Autodesk Inventor part; units mm, degrees
(part 4 of 6)
  line L1347 (22.7558, -15.0073) -> (22.7978, -15.0253) construction
  line L1348 (22.7978, -15.0253) -> (23.0138, -14.7074) construction
  line L1349 (23.0138, -14.7074) -> (23.0378, -14.6833) construction
  spline S408 degree 3 poles (23.0378, -14.6833) (23.0798, -14.6113) (23.1218, -14.5333) (23.1698, -14.4614) knots 110 110 110 110 111 111 111 111
  line L1350 (23.0378, -14.6833) -> (23.0798, -14.6113) construction
  line L1351 (23.0798, -14.6113) -> (23.1218, -14.5333) construction
  line L1352 (23.1218, -14.5333) -> (23.1698, -14.4614) construction
  spline S409 degree 3 poles (23.1698, -14.4614) (23.2118, -14.4073) (23.1998, -14.4134) (23.2598, -14.3894) knots 111 111 111 111 112 112 112 112
  line L1353 (23.1698, -14.4614) -> (23.2118, -14.4073) construction
  line L1354 (23.2118, -14.4073) -> (23.1998, -14.4134) construction
  line L1355 (23.1998, -14.4134) -> (23.2598, -14.3894) construction
  spline S410 degree 3 poles (23.2598, -14.3894) (23.2538, -14.3954) (23.3318, -14.3714) (23.3438, -14.3714) knots 112 112 112 112 113 113 113 113
  line L1356 (23.2598, -14.3894) -> (23.2538, -14.3954) construction
  line L1357 (23.2538, -14.3954) -> (23.3318, -14.3714) construction
  line L1358 (23.3318, -14.3714) -> (23.3438, -14.3714) construction
  spline S411 degree 3 poles (23.3438, -14.3714) (23.3799, -14.3648) (23.6063, -14.3474) (23.7756, -14.2966) knots 113 113 113 113 114 114 114 114
  line L1359 (23.3438, -14.3714) -> (23.3799, -14.3648) construction
  line L1360 (23.3799, -14.3648) -> (23.6063, -14.3474) construction
  line L1361 (23.6063, -14.3474) -> (23.7756, -14.2966) construction
  spline S412 degree 3 poles (23.7756, -14.2966) (23.7091, -14.4879) (23.6088, -14.7871) (23.6258, -14.7913) knots 114 114 114 114 115 115 115 115
  line L1362 (23.7756, -14.2966) -> (23.7091, -14.4879) construction
  line L1363 (23.7091, -14.4879) -> (23.6088, -14.7871) construction
  line L1364 (23.6088, -14.7871) -> (23.6258, -14.7913) construction
  spline S413 degree 3 poles (23.6258, -14.7913) (23.6258, -14.7913) (23.6378, -14.7853) (23.6378, -14.7794) knots 115 115 115 115 116 116 116 116
  line L1365 (23.6258, -14.7913) -> (23.6258, -14.7913) construction
  line L1366 (23.6258, -14.7913) -> (23.6378, -14.7853) construction
  line L1367 (23.6378, -14.7853) -> (23.6378, -14.7794) construction
  spline S414 degree 3 poles (23.6378, -14.7794) (23.6258, -14.8153) (23.6198, -14.8633) (23.6138, -14.9054) knots 116 116 116 116 117 117 117 117
  line L1368 (23.6378, -14.7794) -> (23.6258, -14.8153) construction
  line L1369 (23.6258, -14.8153) -> (23.6198, -14.8633) construction
  line L1370 (23.6198, -14.8633) -> (23.6138, -14.9054) construction
  spline S415 degree 3 poles (23.6138, -14.9054) (23.6018, -14.9054) (23.6198, -14.8693) (23.6078, -14.8693) knots 117 117 117 117 118 118 118 118
  line L1371 (23.6138, -14.9054) -> (23.6018, -14.9054) construction
  line L1372 (23.6018, -14.9054) -> (23.6198, -14.8693) construction
  line L1373 (23.6198, -14.8693) -> (23.6078, -14.8693) construction
  spline S416 degree 3 poles (23.6078, -14.8693) (23.5718, -14.8633) (23.5238, -15.1693) (23.5238, -15.1813) knots 118 118 118 118 119 119 119 119
  line L1374 (23.6078, -14.8693) -> (23.5718, -14.8633) construction
  line L1375 (23.5718, -14.8633) -> (23.5238, -15.1693) construction
  line L1376 (23.5238, -15.1693) -> (23.5238, -15.1813) construction
  spline S417 degree 3 poles (23.5238, -15.1813) (23.5178, -15.3013) (23.5478, -15.4153) (23.6018, -15.5173) knots 119 119 119 119 120 120 120 120
  line L1377 (23.5238, -15.1813) -> (23.5178, -15.3013) construction
  line L1378 (23.5178, -15.3013) -> (23.5478, -15.4153) construction
  line L1379 (23.5478, -15.4153) -> (23.6018, -15.5173) construction
  spline S418 degree 3 poles (23.6018, -15.5173) (23.6438, -15.5833) (23.6858, -15.6373) (23.7578, -15.6613) knots 120 120 120 120 121 121 121 121
  line L1380 (23.6018, -15.5173) -> (23.6438, -15.5833) construction
  line L1381 (23.6438, -15.5833) -> (23.6858, -15.6373) construction
  line L1382 (23.6858, -15.6373) -> (23.7578, -15.6613) construction
  spline S419 degree 3 poles (23.7578, -15.6613) (23.7998, -15.6793) (23.8478, -15.6853) (23.8958, -15.6793) knots 121 121 121 121 122 122 122 122
  line L1383 (23.7578, -15.6613) -> (23.7998, -15.6793) construction
  line L1384 (23.7998, -15.6793) -> (23.8478, -15.6853) construction
  line L1385 (23.8478, -15.6853) -> (23.8958, -15.6793) construction
  spline S420 degree 3 poles (23.8958, -15.6793) (23.9078, -15.6793) (24.0157, -15.6433) (23.9678, -15.6433) knots 122 122 122 122 123 123 123 123
  line L1386 (23.8958, -15.6793) -> (23.9078, -15.6793) construction
  line L1387 (23.9078, -15.6793) -> (24.0157, -15.6433) construction
  line L1388 (24.0157, -15.6433) -> (23.9678, -15.6433) construction
  line L1389 (23.9678, -15.6433) -> (24.0278, -15.6253)
  line L1390 (24.0278, -15.6253) -> (23.9918, -15.6433)
  spline S421 degree 3 poles (23.9918, -15.6433) (23.9978, -15.6493) (24.1658, -15.5653) (24.1898, -15.5593) knots 125 125 125 125 126 126 126 126
  line L1391 (23.9918, -15.6433) -> (23.9978, -15.6493) construction
  line L1392 (23.9978, -15.6493) -> (24.1658, -15.5653) construction
  line L1393 (24.1658, -15.5653) -> (24.1898, -15.5593) construction
  spline S422 degree 3 poles (24.1898, -15.5593) (24.3158, -15.5053) (24.4237, -15.4153) (24.5197, -15.3193) knots 126 126 126 126 127 127 127 127
  line L1394 (24.1898, -15.5593) -> (24.3158, -15.5053) construction
  line L1395 (24.3158, -15.5053) -> (24.4237, -15.4153) construction
  line L1396 (24.4237, -15.4153) -> (24.5197, -15.3193) construction
  spline S423 degree 3 poles (24.5197, -15.3193) (24.7057, -15.1213) (24.8677, -14.8813) (25.0357, -14.6593) knots 127 127 127 127 128 128 128 128
  line L1397 (24.5197, -15.3193) -> (24.7057, -15.1213) construction
  line L1398 (24.7057, -15.1213) -> (24.8677, -14.8813) construction
  line L1399 (24.8677, -14.8813) -> (25.0357, -14.6593) construction
  spline S424 degree 3 poles (25.0357, -14.6593) (25.0237, -14.7253) (24.8737, -15.4753) (24.9157, -15.4753) knots 128 128 128 128 129 129 129 129
  line L1400 (25.0357, -14.6593) -> (25.0237, -14.7253) construction
  line L1401 (25.0237, -14.7253) -> (24.8737, -15.4753) construction
  line L1402 (24.8737, -15.4753) -> (24.9157, -15.4753) construction
  line L1403 (24.9157, -15.4753) -> (24.9277, -15.4513)
  spline S425 degree 3 poles (24.9277, -15.4513) (24.9277, -15.5053) (24.9277, -15.5593) (24.9337, -15.6073) knots 130 130 130 130 131 131 131 131
  line L1404 (24.9277, -15.4513) -> (24.9277, -15.5053) construction
  line L1405 (24.9277, -15.5053) -> (24.9277, -15.5593) construction
  line L1406 (24.9277, -15.5593) -> (24.9337, -15.6073) construction
  spline S426 degree 3 poles (24.9337, -15.6073) (24.9217, -15.6073) (24.9277, -15.5653) (24.9157, -15.5653) knots 131 131 131 131 132 132 132 132
  line L1407 (24.9337, -15.6073) -> (24.9217, -15.6073) construction
  line L1408 (24.9217, -15.6073) -> (24.9277, -15.5653) construction
  line L1409 (24.9277, -15.5653) -> (24.9157, -15.5653) construction
  spline S427 degree 3 poles (24.9157, -15.5653) (24.8797, -15.5713) (24.9217, -15.8233) (24.9277, -15.8473) knots 132 132 132 132 133 133 133 133
  line L1410 (24.9157, -15.5653) -> (24.8797, -15.5713) construction
  line L1411 (24.8797, -15.5713) -> (24.9217, -15.8233) construction
  line L1412 (24.9217, -15.8233) -> (24.9277, -15.8473) construction
  spline S428 degree 3 poles (24.9277, -15.8473) (24.9577, -15.9493) (25.0057, -16.0513) (25.1017, -16.0993) knots 133 133 133 133 134 134 134 134
  line L1413 (24.9277, -15.8473) -> (24.9577, -15.9493) construction
  line L1414 (24.9577, -15.9493) -> (25.0057, -16.0513) construction
  line L1415 (25.0057, -16.0513) -> (25.1017, -16.0993) construction
  spline S429 degree 3 poles (25.1017, -16.0993) (25.1977, -16.1473) (25.3417, -16.1533) (25.4497, -16.1353) knots 134 134 134 134 135 135 135 135
  line L1416 (25.1017, -16.0993) -> (25.1977, -16.1473) construction
  line L1417 (25.1977, -16.1473) -> (25.3417, -16.1533) construction
  line L1418 (25.3417, -16.1533) -> (25.4497, -16.1353) construction
  spline S430 degree 3 poles (25.4497, -16.1353) (25.5217, -16.1233) (25.5997, -16.0933) (25.6597, -16.0453) knots 135 135 135 135 136 136 136 136
  line L1419 (25.4497, -16.1353) -> (25.5217, -16.1233) construction
  line L1420 (25.5217, -16.1233) -> (25.5997, -16.0933) construction
  line L1421 (25.5997, -16.0933) -> (25.6597, -16.0453) construction
  spline S431 degree 3 poles (25.6597, -16.0453) (25.6657, -16.0393) (25.7497, -15.9493) (25.7257, -15.9553) knots 136 136 136 136 137 137 137 137
  line L1422 (25.6597, -16.0453) -> (25.6657, -16.0393) construction
  line L1423 (25.6657, -16.0393) -> (25.7497, -15.9493) construction
  line L1424 (25.7497, -15.9493) -> (25.7257, -15.9553) construction
  line L1425 (25.7257, -15.9553) -> (25.7557, -15.9373)
  spline S432 degree 3 poles (25.7557, -15.9373) (25.7497, -15.9433) (25.7497, -15.9493) (25.7497, -15.9553) knots 138 138 138 138 139 139 139 139
  line L1426 (25.7557, -15.9373) -> (25.7497, -15.9433) construction
  line L1427 (25.7497, -15.9433) -> (25.7497, -15.9493) construction
  line L1428 (25.7497, -15.9493) -> (25.7497, -15.9553) construction
  spline S433 degree 3 poles (25.7497, -15.9553) (25.7557, -15.9613) (25.9357, -15.7693) (25.9597, -15.7513) knots 139 139 139 139 140 140 140 140
  line L1429 (25.7497, -15.9553) -> (25.7557, -15.9613) construction
  line L1430 (25.7557, -15.9613) -> (25.9357, -15.7693) construction
  line L1431 (25.9357, -15.7693) -> (25.9597, -15.7513) construction
  spline S434 degree 3 poles (25.9597, -15.7513) (26.0737, -15.6493) (26.1637, -15.4993) (26.2297, -15.3673) knots 140 140 140 140 141 141 141 141
  line L1432 (25.9597, -15.7513) -> (26.0737, -15.6493) construction
  line L1433 (26.0737, -15.6493) -> (26.1637, -15.4993) construction
  line L1434 (26.1637, -15.4993) -> (26.2297, -15.3673) construction
  line L1435 (26.2297, -15.3673) -> (26.3317, -15.1453)
  line L1436 (26.3317, -15.1453) -> (26.3797, -15.0253)
  spline S435 degree 3 poles (26.3797, -15.0253) (26.3977, -14.9953) (26.4097, -14.9654) (26.4217, -14.9353) knots 143 143 143 143 144 144 144 144
  line L1437 (26.3797, -15.0253) -> (26.3977, -14.9953) construction
  line L1438 (26.3977, -14.9953) -> (26.4097, -14.9654) construction
  line L1439 (26.4097, -14.9654) -> (26.4217, -14.9353) construction
  spline S436 degree 3 poles (26.4217, -14.9353) (26.4337, -14.9353) (26.4517, -14.9413) (26.4637, -14.9413) knots 144 144 144 144 145 145 145 145
  line L1440 (26.4217, -14.9353) -> (26.4337, -14.9353) construction
  line L1441 (26.4337, -14.9353) -> (26.4517, -14.9413) construction
  line L1442 (26.4517, -14.9413) -> (26.4637, -14.9413) construction
  spline S437 degree 3 poles (26.4637, -14.9413) (26.5837, -14.9173) (26.7037, -14.9594) (26.8237, -14.9173) knots 145 145 145 145 146 146 146 146
  line L1443 (26.4637, -14.9413) -> (26.5837, -14.9173) construction
  line L1444 (26.5837, -14.9173) -> (26.7037, -14.9594) construction
  line L1445 (26.7037, -14.9594) -> (26.8237, -14.9173) construction
  spline S438 degree 3 poles (26.8237, -14.9173) (27.0757, -14.8394) (27.2557, -14.6234) (27.4237, -14.4494) knots 146 146 146 146 147 147 147 147
  line L1446 (26.8237, -14.9173) -> (27.0757, -14.8394) construction
  line L1447 (27.0757, -14.8394) -> (27.2557, -14.6234) construction
  line L1448 (27.2557, -14.6234) -> (27.4237, -14.4494) construction
  spline S439 degree 3 poles (27.4237, -14.4494) (27.4717, -14.4013) (27.6337, -14.2694) (27.6217, -14.1734) knots 147 147 147 147 148 148 148 148
  line L1449 (27.4237, -14.4494) -> (27.4717, -14.4013) construction
  line L1450 (27.4717, -14.4013) -> (27.6337, -14.2694) construction
  line L1451 (27.6337, -14.2694) -> (27.6217, -14.1734) construction
  spline S440 degree 3 poles (27.6217, -14.1734) (27.6097, -14.0474) (27.4657, -14.1014) (27.3997, -14.1434) knots 148 148 148 148 149 149 149 149
  line L1452 (27.6217, -14.1734) -> (27.6097, -14.0474) construction
  line L1453 (27.6097, -14.0474) -> (27.4657, -14.1014) construction
  line L1454 (27.4657, -14.1014) -> (27.3997, -14.1434) construction
  spline S441 degree 3 poles (22.6358, -13.2434) (22.6358, -13.2494) (22.6298, -13.2494) (22.6298, -13.2494) knots 0 0 0 0 1 1 1 1
  line L1455 (22.6358, -13.2434) -> (22.6358, -13.2494) construction
  line L1456 (22.6358, -13.2494) -> (22.6298, -13.2494) construction
  line L1457 (22.6298, -13.2494) -> (22.6298, -13.2494) construction
  line L1458 (22.6298, -13.2494) -> (22.6358, -13.2434)
  line L1459 (22.6358, -13.2434) -> (22.6298, -13.2494)
  spline S442 degree 3 poles (22.6298, -13.2494) (22.6298, -13.2494) (22.6358, -13.2494) (22.6358, -13.2434) knots 1 1 1 1 2 2 2 2
  line L1460 (22.6298, -13.2494) -> (22.6298, -13.2494) construction
  line L1461 (22.6298, -13.2494) -> (22.6358, -13.2494) construction
  line L1462 (22.6358, -13.2494) -> (22.6358, -13.2434) construction
  spline S443 degree 3 poles (19.1679, -12.9554) (19.1499, -12.7454) (18.7119, -12.4274) (18.5859, -12.6854) knots 0 0 0 0 1 1 1 1
  line L1463 (19.1679, -12.9554) -> (19.1499, -12.7454) construction
  line L1464 (19.1499, -12.7454) -> (18.7119, -12.4274) construction
  line L1465 (18.7119, -12.4274) -> (18.5859, -12.6854) construction
  spline S444 degree 3 poles (18.5859, -12.6854) (18.5799, -12.6974) (18.5739, -12.7514) (18.5499, -12.7874) knots 1 1 1 1 2 2 2 2
  line L1466 (18.5859, -12.6854) -> (18.5799, -12.6974) construction
  line L1467 (18.5799, -12.6974) -> (18.5739, -12.7514) construction
  line L1468 (18.5739, -12.7514) -> (18.5499, -12.7874) construction
  spline S445 degree 3 poles (18.5499, -12.7874) (18.4839, -12.9014) (18.3879, -13.0094) (18.3039, -13.1174) knots 2 2 2 2 3 3 3 3
  line L1469 (18.5499, -12.7874) -> (18.4839, -12.9014) construction
  line L1470 (18.4839, -12.9014) -> (18.3879, -13.0094) construction
  line L1471 (18.3879, -13.0094) -> (18.3039, -13.1174) construction
  spline S446 degree 3 poles (18.3039, -13.1174) (18.0939, -13.3874) (17.8839, -13.6574) (17.6559, -13.9154) knots 3 3 3 3 4 4 4 4
  line L1472 (18.3039, -13.1174) -> (18.0939, -13.3874) construction
  line L1473 (18.0939, -13.3874) -> (17.8839, -13.6574) construction
  line L1474 (17.8839, -13.6574) -> (17.6559, -13.9154) construction
  line L1475 (17.6559, -13.9154) -> (17.3379, -14.2634)
  spline S447 degree 3 poles (17.3379, -14.2634) (17.3199, -14.2874) (17.0382, -14.5691) (17.0379, -14.5694) knots 5 5 5 5 6 6 6 6
  line L1476 (17.3379, -14.2634) -> (17.3199, -14.2874) construction
  line L1477 (17.3199, -14.2874) -> (17.0379, -14.5694) construction
  line L1478 (17.0379, -14.5694) -> (17.0379, -14.5694) construction
  spline S448 degree 3 poles (17.0379, -14.5694) (17.0619, -14.5814) (17.1339, -14.5094) (17.1519, -14.4974) knots 6 6 6 6 7 7 7 7
  line L1479 (17.0379, -14.5694) -> (17.0619, -14.5814) construction
  line L1480 (17.0619, -14.5814) -> (17.1339, -14.5094) construction
  line L1481 (17.1339, -14.5094) -> (17.1519, -14.4974) construction
  spline S449 degree 3 poles (17.1519, -14.4974) (17.0559, -14.5814) (16.6599, -14.9353) (16.4979, -14.7493) knots 7 7 7 7 8 8 8 8
  line L1482 (17.1519, -14.4974) -> (17.0559, -14.5814) construction
  line L1483 (17.0559, -14.5814) -> (16.6599, -14.9353) construction
  line L1484 (16.6599, -14.9353) -> (16.4979, -14.7493) construction
  spline S450 degree 3 poles (16.4979, -14.7493) (16.3599, -14.5933) (16.5519, -14.2094) (16.6179, -14.0534) knots 8 8 8 8 9 9 9 9
  line L1485 (16.4979, -14.7493) -> (16.3599, -14.5933) construction
  line L1486 (16.3599, -14.5933) -> (16.5519, -14.2094) construction
  line L1487 (16.5519, -14.2094) -> (16.6179, -14.0534) construction
  spline S451 degree 3 poles (16.6179, -14.0534) (16.7259, -13.8014) (16.8399, -13.5434) (16.9659, -13.2974) knots 9 9 9 9 10 10 10 10
  line L1488 (16.6179, -14.0534) -> (16.7259, -13.8014) construction
  line L1489 (16.7259, -13.8014) -> (16.8399, -13.5434) construction
  line L1490 (16.8399, -13.5434) -> (16.9659, -13.2974) construction
  spline S452 degree 3 poles (16.9659, -13.2974) (17.2179, -12.8174) (17.5299, -12.3434) (17.8899, -11.9354) knots 10 10 10 10 11 11 11 11
  line L1491 (16.9659, -13.2974) -> (17.2179, -12.8174) construction
  line L1492 (17.2179, -12.8174) -> (17.5299, -12.3434) construction
  line L1493 (17.5299, -12.3434) -> (17.8899, -11.9354) construction
  spline S453 degree 3 poles (17.8899, -11.9354) (18.0159, -11.7914) (18.2139, -11.5334) (18.4119, -11.4914) knots 11 11 11 11 12 12 12 12
  line L1494 (17.8899, -11.9354) -> (18.0159, -11.7914) construction
  line L1495 (18.0159, -11.7914) -> (18.2139, -11.5334) construction
  line L1496 (18.2139, -11.5334) -> (18.4119, -11.4914) construction
  spline S454 degree 3 poles (18.4119, -11.4914) (18.6459, -11.4434) (18.4419, -11.9294) (18.4719, -11.9354) knots 12 12 12 12 13 13 13 13
  line L1497 (18.4119, -11.4914) -> (18.6459, -11.4434) construction
  line L1498 (18.6459, -11.4434) -> (18.4419, -11.9294) construction
  line L1499 (18.4419, -11.9294) -> (18.4719, -11.9354) construction
  spline S455 degree 3 poles (18.4719, -11.9354) (18.4779, -11.9354) (18.6339, -11.4734) (18.4239, -11.4734) (18.3279, -11.4734) (18.1959, -11.6054) (18.1239, -11.6654) knots 13 13 13 13 14 14 14 15 15 15 15
  line L1500 (18.4719, -11.9354) -> (18.4779, -11.9354) construction
  line L1501 (18.4779, -11.9354) -> (18.6339, -11.4734) construction
  line L1502 (18.6339, -11.4734) -> (18.4239, -11.4734) construction
  line L1503 (18.4239, -11.4734) -> (18.3279, -11.4734) construction
  line L1504 (18.3279, -11.4734) -> (18.1959, -11.6054) construction
  line L1505 (18.1959, -11.6054) -> (18.1239, -11.6654) construction
  spline S456 degree 3 poles (18.1239, -11.6654) (18.0339, -11.7494) (17.9559, -11.8334) (17.8779, -11.9174) knots 15 15 15 15 16 16 16 16
  line L1506 (18.1239, -11.6654) -> (18.0339, -11.7494) construction
  line L1507 (18.0339, -11.7494) -> (17.9559, -11.8334) construction
  line L1508 (17.9559, -11.8334) -> (17.8779, -11.9174) construction
  spline S457 degree 3 poles (17.8779, -11.9174) (18.0399, -11.7374) (18.4239, -11.3114) (18.5259, -11.5214) knots 16 16 16 16 17 17 17 17
  line L1509 (17.8779, -11.9174) -> (18.0399, -11.7374) construction
  line L1510 (18.0399, -11.7374) -> (18.4239, -11.3114) construction
  line L1511 (18.4239, -11.3114) -> (18.5259, -11.5214) construction
  spline S458 degree 3 poles (18.5259, -11.5214) (18.5739, -11.6294) (18.5259, -11.8034) (18.4959, -11.9114) knots 17 17 17 17 18 18 18 18
  line L1512 (18.5259, -11.5214) -> (18.5739, -11.6294) construction
  line L1513 (18.5739, -11.6294) -> (18.5259, -11.8034) construction
  line L1514 (18.5259, -11.8034) -> (18.4959, -11.9114) construction
  spline S459 degree 3 poles (18.4959, -11.9114) (18.4299, -12.1394) (18.3219, -12.3554) (18.1899, -12.5594) knots 18 18 18 18 19 19 19 19
  line L1515 (18.4959, -11.9114) -> (18.4299, -12.1394) construction
  line L1516 (18.4299, -12.1394) -> (18.3219, -12.3554) construction
  line L1517 (18.3219, -12.3554) -> (18.1899, -12.5594) construction
  spline S460 degree 3 poles (18.1899, -12.5594) (18.1959, -12.5474) (18.2858, -12.3796) (18.2859, -12.3794) knots 19 19 19 19 20 20 20 20
  line L1518 (18.1899, -12.5594) -> (18.1959, -12.5474) construction
  line L1519 (18.1959, -12.5474) -> (18.2859, -12.3794) construction
  line L1520 (18.2859, -12.3794) -> (18.2859, -12.3794) construction
  spline S461 degree 3 poles (18.2859, -12.3794) (18.2619, -12.3734) (18.0279, -12.7334) (18.0219, -12.7634) knots 20 20 20 20 21 21 21 21
  line L1521 (18.2859, -12.3794) -> (18.2619, -12.3734) construction
  line L1522 (18.2619, -12.3734) -> (18.0279, -12.7334) construction
  line L1523 (18.0279, -12.7334) -> (18.0219, -12.7634) construction
  spline S462 degree 3 poles (18.0219, -12.7634) (18.0219, -12.7754) (18.0399, -12.7574) (18.0579, -12.7454) knots 21 21 21 21 22 22 22 22
  line L1524 (18.0219, -12.7634) -> (18.0219, -12.7754) construction
  line L1525 (18.0219, -12.7754) -> (18.0399, -12.7574) construction
  line L1526 (18.0399, -12.7574) -> (18.0579, -12.7454) construction
  spline S463 degree 3 poles (18.0579, -12.7454) (18.0219, -12.7934) (18.0099, -12.8294) (18.1239, -12.7994) knots 22 22 22 22 23 23 23 23
  line L1527 (18.0579, -12.7454) -> (18.0219, -12.7934) construction
  line L1528 (18.0219, -12.7934) -> (18.0099, -12.8294) construction
  line L1529 (18.0099, -12.8294) -> (18.1239, -12.7994) construction
  spline S464 degree 3 poles (18.1239, -12.7994) (18.3219, -12.7454) (18.5439, -12.5474) (18.6879, -12.4094) knots 23 23 23 23 24 24 24 24
  line L1530 (18.1239, -12.7994) -> (18.3219, -12.7454) construction
  line L1531 (18.3219, -12.7454) -> (18.5439, -12.5474) construction
  line L1532 (18.5439, -12.5474) -> (18.6879, -12.4094) construction
  spline S465 degree 3 poles (18.6879, -12.4094) (18.8379, -12.2654) (19.0179, -12.0614) (19.0119, -11.8454) knots 24 24 24 24 25 25 25 25
  line L1533 (18.6879, -12.4094) -> (18.8379, -12.2654) construction
  line L1534 (18.8379, -12.2654) -> (19.0179, -12.0614) construction
  line L1535 (19.0179, -12.0614) -> (19.0119, -11.8454) construction
  spline S466 degree 3 poles (19.0119, -11.8454) (19.0119, -11.7614) (18.9699, -11.7014) (18.9639, -11.6234) knots 25 25 25 25 26 26 26 26
  line L1536 (19.0119, -11.8454) -> (19.0119, -11.7614) construction
  line L1537 (19.0119, -11.7614) -> (18.9699, -11.7014) construction
  line L1538 (18.9699, -11.7014) -> (18.9639, -11.6234) construction
  spline S467 degree 3 poles (18.9639, -11.6234) (18.9519, -11.5394) (18.9519, -11.4794) (18.8979, -11.3954) knots 26 26 26 26 27 27 27 27
  line L1539 (18.9639, -11.6234) -> (18.9519, -11.5394) construction
  line L1540 (18.9519, -11.5394) -> (18.9519, -11.4794) construction
  line L1541 (18.9519, -11.4794) -> (18.8979, -11.3954) construction
  spline S468 degree 3 poles (18.8979, -11.3954) (18.7419, -11.1554) (18.4779, -10.9874) (18.1899, -11.0294) knots 27 27 27 27 28 28 28 28
  line L1542 (18.8979, -11.3954) -> (18.7419, -11.1554) construction
  line L1543 (18.7419, -11.1554) -> (18.4779, -10.9874) construction
  line L1544 (18.4779, -10.9874) -> (18.1899, -11.0294) construction
  spline S469 degree 3 poles (18.1899, -11.0294) (17.9319, -11.0594) (17.7159, -11.2394) (17.5359, -11.4134) knots 28 28 28 28 29 29 29 29
  line L1545 (18.1899, -11.0294) -> (17.9319, -11.0594) construction
  line L1546 (17.9319, -11.0594) -> (17.7159, -11.2394) construction
  line L1547 (17.7159, -11.2394) -> (17.5359, -11.4134) construction
  spline S470 degree 3 poles (17.5359, -11.4134) (17.4399, -11.5094) (17.3559, -11.6114) (17.2659, -11.7134) knots 29 29 29 29 30 30 30 30
  line L1548 (17.5359, -11.4134) -> (17.4399, -11.5094) construction
  line L1549 (17.4399, -11.5094) -> (17.3559, -11.6114) construction
  line L1550 (17.3559, -11.6114) -> (17.2659, -11.7134) construction
  spline S471 degree 3 poles (17.2659, -11.7134) (17.2059, -11.7854) (17.0739, -11.8874) (17.0499, -11.9834) knots 30 30 30 30 31 31 31 31
  line L1551 (17.2659, -11.7134) -> (17.2059, -11.7854) construction
  line L1552 (17.2059, -11.7854) -> (17.0739, -11.8874) construction
  line L1553 (17.0739, -11.8874) -> (17.0499, -11.9834) construction
  line L1554 (17.0499, -11.9834) -> (17.0979, -11.9354)
  spline S472 degree 3 poles (17.0979, -11.9354) (17.0259, -12.0254) (16.9659, -12.1214) (16.9119, -12.1934) knots 32 32 32 32 33 33 33 33
  line L1555 (17.0979, -11.9354) -> (17.0259, -12.0254) construction
  line L1556 (17.0259, -12.0254) -> (16.9659, -12.1214) construction
  line L1557 (16.9659, -12.1214) -> (16.9119, -12.1934) construction
  spline S473 degree 3 poles (16.9119, -12.1934) (16.9059, -12.1934) (16.9479, -12.1215) (16.9479, -12.1214) knots 33 33 33 33 34 34 34 34
  line L1558 (16.9119, -12.1934) -> (16.9059, -12.1934) construction
  line L1559 (16.9059, -12.1934) -> (16.9479, -12.1214) construction
  line L1560 (16.9479, -12.1214) -> (16.9479, -12.1214) construction
  spline S474 degree 3 poles (16.9479, -12.1214) (16.9059, -12.1034) (16.6599, -12.4994) (16.6359, -12.5354) knots 34 34 34 34 35 35 35 35
  line L1561 (16.9479, -12.1214) -> (16.9059, -12.1034) construction
  line L1562 (16.9059, -12.1034) -> (16.6599, -12.4994) construction
  line L1563 (16.6599, -12.4994) -> (16.6359, -12.5354) construction
  spline S475 degree 3 poles (16.6359, -12.5354) (16.5219, -12.7094) (16.4199, -12.8834) (16.3479, -13.0754) (16.2759, -13.2674) (16.1859, -13.4594) (16.1139, -13.6514) knots 35 35 35 35 36 36 36 37 37 37 37
  line L1564 (16.6359, -12.5354) -> (16.5219, -12.7094) construction
  line L1565 (16.5219, -12.7094) -> (16.4199, -12.8834) construction
  line L1566 (16.4199, -12.8834) -> (16.3479, -13.0754) construction
  line L1567 (16.3479, -13.0754) -> (16.2759, -13.2674) construction
  line L1568 (16.2759, -13.2674) -> (16.1859, -13.4594) construction
  line L1569 (16.1859, -13.4594) -> (16.1139, -13.6514) construction
  spline S476 degree 3 poles (16.1139, -13.6514) (16.0659, -13.7714) (16.0299, -13.8914) (15.9999, -14.0114) knots 37 37 37 37 38 38 38 38
  line L1570 (16.1139, -13.6514) -> (16.0659, -13.7714) construction
  line L1571 (16.0659, -13.7714) -> (16.0299, -13.8914) construction
  line L1572 (16.0299, -13.8914) -> (15.9999, -14.0114) construction
  spline S477 degree 3 poles (15.9999, -14.0114) (15.9939, -14.0474) (15.991, -14.2274) (16.009, -14.1974) knots 38 38 38 38 39 39 39 39
  line L1573 (15.9999, -14.0114) -> (15.9939, -14.0474) construction
  line L1574 (15.9939, -14.0474) -> (15.991, -14.2274) construction
  line L1575 (15.991, -14.2274) -> (16.009, -14.1974) construction
  line L1576 (16.009, -14.1974) -> (16, -14.3354)
  line L1577 (16, -14.3354) -> (16, -14.2274)
  spline S478 degree 3 poles (16, -14.2274) (15.9583, -14.2514) (15.991, -14.3714) (15.991, -14.3774) knots 41 41 41 41 42 42 42 42
  line L1578 (16, -14.2274) -> (15.9583, -14.2514) construction
  line L1579 (15.9583, -14.2514) -> (15.991, -14.3714) construction
  line L1580 (15.991, -14.3714) -> (15.991, -14.3774) construction
  spline S479 degree 3 poles (15.991, -14.3774) (15.979, -14.7734) (16.3464, -15.3433) (16.7964, -15.2893) knots 42 42 42 42 43 43 43 43
  line L1581 (15.991, -14.3774) -> (15.979, -14.7734) construction
  line L1582 (15.979, -14.7734) -> (16.3464, -15.3433) construction
  line L1583 (16.3464, -15.3433) -> (16.7964, -15.2893) construction
  spline S480 degree 3 poles (16.7964, -15.2893) (17.0604, -15.2593) (17.2742, -15.0193) (17.4422, -14.8334) knots 43 43 43 43 44 44 44 44
  line L1584 (16.7964, -15.2893) -> (17.0604, -15.2593) construction
  line L1585 (17.0604, -15.2593) -> (17.2742, -15.0193) construction
  line L1586 (17.2742, -15.0193) -> (17.4422, -14.8334) construction
  spline S481 degree 3 poles (17.4422, -14.8334) (17.7062, -14.5273) (17.945, -14.1854) (18.155, -13.8374) knots 44 44 44 44 45 45 45 45
  line L1587 (17.4422, -14.8334) -> (17.7062, -14.5273) construction
  line L1588 (17.7062, -14.5273) -> (17.945, -14.1854) construction
  line L1589 (17.945, -14.1854) -> (18.155, -13.8374) construction
  spline S482 degree 3 poles (18.155, -13.8374) (17.939, -14.4494) (17.7345, -15.0613) (17.5005, -15.6613) knots 45 45 45 45 46 46 46 46
  line L1590 (18.155, -13.8374) -> (17.939, -14.4494) construction
  line L1591 (17.939, -14.4494) -> (17.7345, -15.0613) construction
  line L1592 (17.7345, -15.0613) -> (17.5005, -15.6613) construction
  spline S483 degree 3 poles (17.5005, -15.6613) (17.2665, -16.2433) (17.0322, -16.8613) (16.6602, -17.3713) knots 46 46 46 46 47 47 47 47
  line L1593 (17.5005, -15.6613) -> (17.2665, -16.2433) construction
  line L1594 (17.2665, -16.2433) -> (17.0322, -16.8613) construction
  line L1595 (17.0322, -16.8613) -> (16.6602, -17.3713) construction
  spline S484 degree 3 poles (16.6602, -17.3713) (16.5642, -17.4973) (16.3361, -17.7673) (16.1741, -17.5813) knots 47 47 47 47 48 48 48 48
  line L1596 (16.6602, -17.3713) -> (16.5642, -17.4973) construction
  line L1597 (16.5642, -17.4973) -> (16.3361, -17.7673) construction
  line L1598 (16.3361, -17.7673) -> (16.1741, -17.5813) construction
  spline S485 degree 3 poles (16.1741, -17.5813) (16.0001, -17.3893) (16.246, -16.9333) (16.336, -16.7533) knots 48 48 48 48 49 49 49 49
  line L1599 (16.1741, -17.5813) -> (16.0001, -17.3893) construction
  line L1600 (16.0001, -17.3893) -> (16.246, -16.9333) construction
  line L1601 (16.246, -16.9333) -> (16.336, -16.7533) construction
  spline S486 degree 3 poles (16.336, -16.7533) (16.468, -16.4713) (16.636, -16.2073) (16.828, -15.9673) knots 49 49 49 49 50 50 50 50
  line L1602 (16.336, -16.7533) -> (16.468, -16.4713) construction
  line L1603 (16.468, -16.4713) -> (16.636, -16.2073) construction
  line L1604 (16.636, -16.2073) -> (16.828, -15.9673) construction
  spline S487 degree 3 poles (16.828, -15.9673) (16.858, -15.9313) (17.1459, -15.6553) (16.9599, -15.6673) knots 50 50 50 50 51 51 51 51
  line L1605 (16.828, -15.9673) -> (16.858, -15.9313) construction
  line L1606 (16.858, -15.9313) -> (17.1459, -15.6553) construction
  line L1607 (17.1459, -15.6553) -> (16.9599, -15.6673) construction
  spline S488 degree 3 poles (16.9599, -15.6673) (16.8699, -15.6733) (16.7619, -15.8053) (16.7019, -15.8593) knots 51 51 51 51 52 52 52 52
  line L1608 (16.9599, -15.6673) -> (16.8699, -15.6733) construction
  line L1609 (16.8699, -15.6733) -> (16.7619, -15.8053) construction
  line L1610 (16.7619, -15.8053) -> (16.7019, -15.8593) construction
  spline S489 degree 3 poles (16.7019, -15.8593) (16.6179, -15.9313) (16.5399, -16.0153) (16.4499, -16.0813) knots 52 52 52 52 53 53 53 53
  line L1611 (16.7019, -15.8593) -> (16.6179, -15.9313) construction
  line L1612 (16.6179, -15.9313) -> (16.5399, -16.0153) construction
  line L1613 (16.5399, -16.0153) -> (16.4499, -16.0813) construction
  spline S490 degree 3 poles (16.4499, -16.0813) (16.2159, -16.2733) (16.0059, -16.5073) (15.8559, -16.7713) knots 53 53 53 53 54 54 54 54
  line L1614 (16.4499, -16.0813) -> (16.2159, -16.2733) construction
  line L1615 (16.2159, -16.2733) -> (16.0059, -16.5073) construction
  line L1616 (16.0059, -16.5073) -> (15.8559, -16.7713) construction
  spline S491 degree 3 poles (15.8559, -16.7713) (15.6099, -17.2153) (15.6579, -17.7373) (16.1739, -17.9533) knots 54 54 54 54 55 55 55 55
  line L1617 (15.8559, -16.7713) -> (15.6099, -17.2153) construction
  line L1618 (15.6099, -17.2153) -> (15.6579, -17.7373) construction
  line L1619 (15.6579, -17.7373) -> (16.1739, -17.9533) construction
  spline S492 degree 3 poles (16.1739, -17.9533) (16.3299, -18.0193) (16.5399, -18.0733) (16.7019, -18.0013) knots 55 55 55 55 56 56 56 56
  line L1620 (16.1739, -17.9533) -> (16.3299, -18.0193) construction
  line L1621 (16.3299, -18.0193) -> (16.5399, -18.0733) construction
  line L1622 (16.5399, -18.0733) -> (16.7019, -18.0013) construction
  spline S493 degree 3 poles (16.7019, -18.0013) (16.8639, -17.9293) (17.0019, -17.7493) (17.1039, -17.6113) knots 56 56 56 56 57 57 57 57
  line L1623 (16.7019, -18.0013) -> (16.8639, -17.9293) construction
  line L1624 (16.8639, -17.9293) -> (17.0019, -17.7493) construction
  line L1625 (17.0019, -17.7493) -> (17.1039, -17.6113) construction
  spline S494 degree 3 poles (17.1039, -17.6113) (17.2959, -17.3653) (17.4219, -17.0893) (17.5659, -16.8133) knots 57 57 57 57 58 58 58 58
  line L1626 (17.1039, -17.6113) -> (17.2959, -17.3653) construction
  line L1627 (17.2959, -17.3653) -> (17.4219, -17.0893) construction
  line L1628 (17.4219, -17.0893) -> (17.5659, -16.8133) construction
  spline S495 degree 3 poles (17.5659, -16.8133) (17.7039, -16.5553) (17.8659, -16.2853) (17.9439, -15.9973) knots 58 58 58 58 59 59 59 59
  line L1629 (17.5659, -16.8133) -> (17.7039, -16.5553) construction
  line L1630 (17.7039, -16.5553) -> (17.8659, -16.2853) construction
  line L1631 (17.8659, -16.2853) -> (17.9439, -15.9973) construction
  spline S496 degree 3 poles (17.9439, -15.9973) (18.0219, -15.7213) (18.1659, -15.4573) (18.2739, -15.1813) knots 59 59 59 59 60 60 60 60
  line L1632 (17.9439, -15.9973) -> (18.0219, -15.7213) construction
  line L1633 (18.0219, -15.7213) -> (18.1659, -15.4573) construction
  line L1634 (18.1659, -15.4573) -> (18.2739, -15.1813) construction
  line L1635 (18.2739, -15.1813) -> (18.6339, -14.2994)
  spline S497 degree 3 poles (18.6339, -14.2994) (18.6939, -14.1314) (18.7719, -13.9694) (18.8259, -13.8074) knots 61 61 61 61 62 62 62 62
  line L1636 (18.6339, -14.2994) -> (18.6939, -14.1314) construction
  line L1637 (18.6939, -14.1314) -> (18.7719, -13.9694) construction
  line L1638 (18.7719, -13.9694) -> (18.8259, -13.8074) construction
  spline S498 degree 3 poles (18.8259, -13.8074) (18.8619, -13.7114) (18.8499, -13.6514) (18.8919, -13.5674) knots 62 62 62 62 63 63 63 63
  line L1639 (18.8259, -13.8074) -> (18.8619, -13.7114) construction
  line L1640 (18.8619, -13.7114) -> (18.8499, -13.6514) construction
  line L1641 (18.8499, -13.6514) -> (18.8919, -13.5674) construction
  spline S499 degree 3 poles (18.8919, -13.5674) (18.9699, -13.4234) (19.0479, -13.2794) (19.1199, -13.1354) knots 63 63 63 63 64 64 64 64
  line L1642 (18.8919, -13.5674) -> (18.9699, -13.4234) construction
  line L1643 (18.9699, -13.4234) -> (19.0479, -13.2794) construction
  line L1644 (19.0479, -13.2794) -> (19.1199, -13.1354) construction
  spline S500 degree 3 poles (19.1199, -13.1354) (19.1499, -13.0754) (19.1739, -13.0214) (19.1679, -12.9554) knots 64 64 64 64 65 65 65 65
  line L1645 (19.1199, -13.1354) -> (19.1499, -13.0754) construction
  line L1646 (19.1499, -13.0754) -> (19.1739, -13.0214) construction
  line L1647 (19.1739, -13.0214) -> (19.1679, -12.9554) construction
  line L1648 (14.4583, -14.1014) -> (14.4583, -14.0954)
  spline S501 degree 3 poles (14.4583, -14.0954) (14.375, -13.9334) (14.2362, -14.1554) (14.1821, -14.2334) knots 1 1 1 1 2 2 2 2
  line L1649 (14.4583, -14.0954) -> (14.375, -13.9334) construction
  line L1650 (14.375, -13.9334) -> (14.2362, -14.1554) construction
  line L1651 (14.2362, -14.1554) -> (14.1821, -14.2334) construction
  spline S502 degree 3 poles (14.1821, -14.2334) (14.0802, -14.3714) (13.9841, -14.5034) (13.8761, -14.6294) knots 2 2 2 2 3 3 3 3
  line L1652 (14.1821, -14.2334) -> (14.0802, -14.3714) construction
  line L1653 (14.0802, -14.3714) -> (13.9841, -14.5034) construction
  line L1654 (13.9841, -14.5034) -> (13.8761, -14.6294) construction
  spline S503 degree 3 poles (13.8761, -14.6294) (13.7861, -14.7373) (13.69, -14.8454) (13.618, -14.9594) knots 3 3 3 3 4 4 4 4
  line L1655 (13.8761, -14.6294) -> (13.7861, -14.7373) construction
  line L1656 (13.7861, -14.7373) -> (13.69, -14.8454) construction
  line L1657 (13.69, -14.8454) -> (13.618, -14.9594) construction
  spline S504 degree 3 poles (13.618, -14.9594) (13.618, -14.9714) (13.606, -15.0013) (13.606, -15.0013) knots 4 4 4 4 5 5 5 5
  line L1658 (13.618, -14.9594) -> (13.618, -14.9714) construction
  line L1659 (13.618, -14.9714) -> (13.606, -15.0013) construction
  line L1660 (13.606, -15.0013) -> (13.606, -15.0013) construction
  spline S505 degree 3 poles (13.606, -15.0013) (13.582, -15.0374) (13.546, -15.0673) (13.516, -15.1034) knots 5 5 5 5 6 6 6 6
  line L1661 (13.606, -15.0013) -> (13.582, -15.0374) construction
  line L1662 (13.582, -15.0374) -> (13.546, -15.0673) construction
  line L1663 (13.546, -15.0673) -> (13.516, -15.1034) construction
  spline S506 degree 3 poles (13.516, -15.1034) (13.462, -15.1573) (13.408, -15.2173) (13.348, -15.2713) knots 6 6 6 6 7 7 7 7
  line L1664 (13.516, -15.1034) -> (13.462, -15.1573) construction
  line L1665 (13.462, -15.1573) -> (13.408, -15.2173) construction
  line L1666 (13.408, -15.2173) -> (13.348, -15.2713) construction
  spline S507 degree 3 poles (13.348, -15.2713) (13.258, -15.3553) (12.754, -15.8293) (12.688, -15.5233) knots 7 7 7 7 8 8 8 8
  line L1667 (13.348, -15.2713) -> (13.258, -15.3553) construction
  line L1668 (13.258, -15.3553) -> (12.754, -15.8293) construction
  line L1669 (12.754, -15.8293) -> (12.688, -15.5233) construction
  spline S508 degree 3 poles (12.688, -15.5233) (12.652, -15.3733) (12.7, -15.1873) (12.73, -15.0433) knots 8 8 8 8 9 9 9 9
  line L1670 (12.688, -15.5233) -> (12.652, -15.3733) construction
  line L1671 (12.652, -15.3733) -> (12.7, -15.1873) construction
  line L1672 (12.7, -15.1873) -> (12.73, -15.0433) construction
  spline S509 degree 3 poles (12.73, -15.0433) (12.748, -14.9654) (12.766, -14.8934) (12.778, -14.8153) knots 9 9 9 9 10 10 10 10
  line L1673 (12.73, -15.0433) -> (12.748, -14.9654) construction
  line L1674 (12.748, -14.9654) -> (12.766, -14.8934) construction
  line L1675 (12.766, -14.8934) -> (12.778, -14.8153) construction
  spline S510 degree 3 poles (12.778, -14.8153) (12.79, -14.7554) (12.772, -14.6954) (12.802, -14.6354) knots 10 10 10 10 11 11 11 11
  line L1676 (12.778, -14.8153) -> (12.79, -14.7554) construction
  line L1677 (12.79, -14.7554) -> (12.772, -14.6954) construction
  line L1678 (12.772, -14.6954) -> (12.802, -14.6354) construction
  spline S511 degree 3 poles (12.802, -14.6354) (12.82, -14.5993) (12.826, -14.6053) (12.868, -14.5933) knots 11 11 11 11 12 12 12 12
  line L1679 (12.802, -14.6354) -> (12.82, -14.5993) construction
  line L1680 (12.82, -14.5993) -> (12.826, -14.6053) construction
  line L1681 (12.826, -14.6053) -> (12.868, -14.5933) construction
  line L1682 (12.868, -14.5933) -> (12.97, -14.5574)
  spline S512 degree 3 poles (12.97, -14.5574) (13.036, -14.5333) (13.102, -14.5094) (13.162, -14.4733) knots 13 13 13 13 14 14 14 14
  line L1683 (12.97, -14.5574) -> (13.036, -14.5333) construction
  line L1684 (13.036, -14.5333) -> (13.102, -14.5094) construction
  line L1685 (13.102, -14.5094) -> (13.162, -14.4733) construction
  spline S513 degree 3 poles (13.162, -14.4733) (13.252, -14.4194) (13.336, -14.3534) (13.414, -14.2874) knots 14 14 14 14 15 15 15 15
  line L1686 (13.162, -14.4733) -> (13.252, -14.4194) construction
  line L1687 (13.252, -14.4194) -> (13.336, -14.3534) construction
  line L1688 (13.336, -14.3534) -> (13.414, -14.2874) construction
  spline S514 degree 3 poles (13.414, -14.2874) (13.6, -14.1314) (13.798, -13.9454) (13.876, -13.7114) knots 15 15 15 15 16 16 16 16
  line L1689 (13.414, -14.2874) -> (13.6, -14.1314) construction
  line L1690 (13.6, -14.1314) -> (13.798, -13.9454) construction
  line L1691 (13.798, -13.9454) -> (13.876, -13.7114) construction
  spline S515 degree 3 poles (13.876, -13.7114) (13.918, -13.5794) (13.924, -13.4354) (13.84, -13.3214) knots 16 16 16 16 17 17 17 17
  line L1692 (13.876, -13.7114) -> (13.918, -13.5794) construction
  line L1693 (13.918, -13.5794) -> (13.924, -13.4354) construction
  line L1694 (13.924, -13.4354) -> (13.84, -13.3214) construction
  spline S516 degree 3 poles (13.84, -13.3214) (13.762, -13.2194) (13.63, -13.1654) (13.51, -13.1414) knots 17 17 17 17 18 18 18 18
  line L1695 (13.84, -13.3214) -> (13.762, -13.2194) construction
  line L1696 (13.762, -13.2194) -> (13.63, -13.1654) construction
  line L1697 (13.63, -13.1654) -> (13.51, -13.1414) construction
  spline S517 degree 3 poles (13.51, -13.1414) (13.186, -13.0814) (12.94, -13.2674) (12.754, -13.5134) knots 18 18 18 18 19 19 19 19
  line L1698 (13.51, -13.1414) -> (13.186, -13.0814) construction
  line L1699 (13.186, -13.0814) -> (12.94, -13.2674) construction
  line L1700 (12.94, -13.2674) -> (12.754, -13.5134) construction
  spline S518 degree 3 poles (12.754, -13.5134) (12.6166, -13.6833) (12.5038, -13.8773) (12.4183, -14.082) knots 19 19 19 19 20 20 20 20
  line L1701 (12.754, -13.5134) -> (12.6166, -13.6833) construction
  line L1702 (12.6166, -13.6833) -> (12.5038, -13.8773) construction
  line L1703 (12.5038, -13.8773) -> (12.4183, -14.082) construction
  spline S519 degree 3 poles (12.4183, -14.082) (12.3475, -14.1729) (12.2975, -14.304) (12.238, -14.4013) knots 20 20 20 20 21 21 21 21
  line L1704 (12.4183, -14.082) -> (12.3475, -14.1729) construction
  line L1705 (12.3475, -14.1729) -> (12.2975, -14.304) construction
  line L1706 (12.2975, -14.304) -> (12.238, -14.4013) construction
  spline S520 degree 3 poles (12.238, -14.4013) (12.136, -14.5754) (12.034, -14.7433) (11.926, -14.9113) knots 21 21 21 21 22 22 22 22
  line L1707 (12.238, -14.4013) -> (12.136, -14.5754) construction
  line L1708 (12.136, -14.5754) -> (12.034, -14.7433) construction
  line L1709 (12.034, -14.7433) -> (11.926, -14.9113) construction
  spline S521 degree 3 poles (11.926, -14.9113) (11.722, -15.2353) (11.518, -15.5653) (11.2721, -15.8593) knots 22 22 22 22 23 23 23 23
  line L1710 (11.926, -14.9113) -> (11.722, -15.2353) construction
  line L1711 (11.722, -15.2353) -> (11.518, -15.5653) construction
  line L1712 (11.518, -15.5653) -> (11.2721, -15.8593) construction
  spline S522 degree 3 poles (11.2721, -15.8593) (11.17, -15.9853) (10.9541, -16.2913) (10.7501, -16.2673) knots 23 23 23 23 24 24 24 24
  line L1713 (11.2721, -15.8593) -> (11.17, -15.9853) construction
  line L1714 (11.17, -15.9853) -> (10.9541, -16.2913) construction
  line L1715 (10.9541, -16.2913) -> (10.7501, -16.2673) construction
  spline S523 degree 3 poles (10.7501, -16.2673) (10.6001, -16.2433) (10.6001, -15.9853) (10.6001, -15.8713) (10.6001, -15.7753) (10.6061, -15.6793) (10.6181, -15.5893) knots 24 24 24 24 25 25 25 26 26 26 26
  line L1716 (10.7501, -16.2673) -> (10.6001, -16.2433) construction
  line L1717 (10.6001, -16.2433) -> (10.6001, -15.9853) construction
  line L1718 (10.6001, -15.9853) -> (10.6001, -15.8713) construction
  line L1719 (10.6001, -15.8713) -> (10.6001, -15.7753) construction
  line L1720 (10.6001, -15.7753) -> (10.6061, -15.6793) construction
  line L1721 (10.6061, -15.6793) -> (10.6181, -15.5893) construction
  spline S524 degree 3 poles (10.6181, -15.5893) (10.6241, -15.5353) (10.6721, -15.3553) (10.6421, -15.3073) knots 26 26 26 26 27 27 27 27
  line L1722 (10.6181, -15.5893) -> (10.6241, -15.5353) construction
  line L1723 (10.6241, -15.5353) -> (10.6721, -15.3553) construction
  line L1724 (10.6721, -15.3553) -> (10.6421, -15.3073) construction
  line L1725 (10.6421, -15.3073) -> (10.5941, -15.4873)
  spline S525 degree 3 poles (10.5941, -15.4873) (10.6001, -15.4153) (10.6121, -15.3373) (10.6301, -15.2653) knots 28 28 28 28 29 29 29 29
  line L1726 (10.5941, -15.4873) -> (10.6001, -15.4153) construction
  line L1727 (10.6001, -15.4153) -> (10.6121, -15.3373) construction
  line L1728 (10.6121, -15.3373) -> (10.6301, -15.2653) construction
  spline S526 degree 3 poles (10.6301, -15.2653) (10.6241, -15.2533) (10.6781, -15.0853) (10.6901, -15.0314) knots 29 29 29 29 30 30 30 30
  line L1729 (10.6301, -15.2653) -> (10.6241, -15.2533) construction
  line L1730 (10.6241, -15.2533) -> (10.6781, -15.0853) construction
  line L1731 (10.6781, -15.0853) -> (10.6901, -15.0314) construction
  spline S527 degree 3 poles (10.6901, -15.0314) (10.7201, -14.9113) (10.7501, -14.7913) (10.7861, -14.6713) knots 30 30 30 30 31 31 31 31
  line L1732 (10.6901, -15.0314) -> (10.7201, -14.9113) construction
  line L1733 (10.7201, -14.9113) -> (10.7501, -14.7913) construction
  line L1734 (10.7501, -14.7913) -> (10.7861, -14.6713) construction
  spline S528 degree 3 poles (10.7861, -14.6713) (10.8161, -14.5514) (10.846, -14.4374) (10.8821, -14.3234) knots 31 31 31 31 32 32 32 32
  line L1735 (10.7861, -14.6713) -> (10.8161, -14.5514) construction
  line L1736 (10.8161, -14.5514) -> (10.846, -14.4374) construction
  line L1737 (10.846, -14.4374) -> (10.8821, -14.3234) construction
  spline S529 degree 3 poles (10.8821, -14.3234) (10.912, -14.2154) (10.9541, -14.1614) (11.0201, -14.0774) knots 32 32 32 32 33 33 33 33
  line L1738 (10.8821, -14.3234) -> (10.912, -14.2154) construction
  line L1739 (10.912, -14.2154) -> (10.9541, -14.1614) construction
  line L1740 (10.9541, -14.1614) -> (11.0201, -14.0774) construction
  spline S530 degree 3 poles (11.0201, -14.0774) (11.29, -13.7414) (11.5361, -13.3754) (11.764, -13.0094) knots 33 33 33 33 34 34 34 34
  line L1741 (11.0201, -14.0774) -> (11.29, -13.7414) construction
  line L1742 (11.29, -13.7414) -> (11.5361, -13.3754) construction
  line L1743 (11.5361, -13.3754) -> (11.764, -13.0094) construction
  spline S531 degree 3 poles (11.764, -13.0094) (11.848, -12.8714) (11.902, -12.7514) (12.004, -12.6374) knots 34 34 34 34 35 35 35 35
  line L1744 (11.764, -13.0094) -> (11.848, -12.8714) construction
  line L1745 (11.848, -12.8714) -> (11.902, -12.7514) construction
  line L1746 (11.902, -12.7514) -> (12.004, -12.6374) construction
  spline S532 degree 3 poles (12.004, -12.6374) (12.154, -12.4814) (12.2632, -12.2474) (12.3592, -12.0554) knots 35 35 35 35 36 36 36 36
  line L1747 (12.004, -12.6374) -> (12.154, -12.4814) construction
  line L1748 (12.154, -12.4814) -> (12.2632, -12.2474) construction
  line L1749 (12.2632, -12.2474) -> (12.3592, -12.0554) construction
  spline S533 degree 3 poles (12.3592, -12.0554) (12.5212, -11.7434) (12.75, -11.3114) (12.7083, -10.9454) knots 36 36 36 36 37 37 37 37
  line L1750 (12.3592, -12.0554) -> (12.5212, -11.7434) construction
  line L1751 (12.5212, -11.7434) -> (12.75, -11.3114) construction
  line L1752 (12.75, -11.3114) -> (12.7083, -10.9454) construction
  line L1753 (12.7083, -10.9454) -> (12.7083, -10.9154)
  line L1754 (12.7083, -10.9154) -> (12.6952, -10.9094)
  spline S534 degree 3 poles (12.6952, -10.9094) (12.6592, -10.6754) (12.4396, -10.3994) (12.1756, -10.4834) knots 39 39 39 39 40 40 40 40
  line L1755 (12.6952, -10.9094) -> (12.6592, -10.6754) construction
  line L1756 (12.6592, -10.6754) -> (12.4396, -10.3994) construction
  line L1757 (12.4396, -10.3994) -> (12.1756, -10.4834) construction
  spline S535 degree 3 poles (12.1756, -10.4834) (12.0376, -10.5254) (11.9338, -10.6694) (11.8498, -10.7714) knots 40 40 40 40 41 41 41 41
  line L1758 (12.1756, -10.4834) -> (12.0376, -10.5254) construction
  line L1759 (12.0376, -10.5254) -> (11.9338, -10.6694) construction
  line L1760 (11.9338, -10.6694) -> (11.8498, -10.7714) construction
  line L1761 (11.8498, -10.7714) -> (11.7109, -10.9574)
  spline S536 degree 3 poles (11.7109, -10.9574) (11.6809, -10.9934) (11.6385, -11.0834) (11.6085, -11.1314) knots 42 42 42 42 43 43 43 43
  line L1762 (11.7109, -10.9574) -> (11.6809, -10.9934) construction
  line L1763 (11.6809, -10.9934) -> (11.6385, -11.0834) construction
  line L1764 (11.6385, -11.0834) -> (11.6085, -11.1314) construction
  line L1765 (11.6085, -11.1314) -> (11.6143, -11.1254)
  line L1766 (11.6143, -11.1254) -> (11.4222, -11.4554)
  line L1767 (11.4222, -11.4554) -> (11.4701, -11.3534)
  spline S537 degree 3 poles (11.4701, -11.3534) (11.4401, -11.3474) (11.3081, -11.6054) (11.2901, -11.6354) knots 46 46 46 46 47 47 47 47
  line L1768 (11.4701, -11.3534) -> (11.4401, -11.3474) construction
  line L1769 (11.4401, -11.3474) -> (11.3081, -11.6054) construction
  line L1770 (11.3081, -11.6054) -> (11.2901, -11.6354) construction
  spline S538 degree 3 poles (11.2901, -11.6354) (11.2241, -11.7494) (11.1641, -11.8634) (11.1101, -11.9774) knots 47 47 47 47 48 48 48 48
  line L1771 (11.2901, -11.6354) -> (11.2241, -11.7494) construction
  line L1772 (11.2241, -11.7494) -> (11.1641, -11.8634) construction
  line L1773 (11.1641, -11.8634) -> (11.1101, -11.9774) construction
  spline S539 degree 3 poles (11.1101, -11.9774) (10.9901, -12.2174) (10.8701, -12.4634) (10.7921, -12.7214) knots 48 48 48 48 49 49 49 49
  line L1774 (11.1101, -11.9774) -> (10.9901, -12.2174) construction
  line L1775 (10.9901, -12.2174) -> (10.8701, -12.4634) construction
  line L1776 (10.8701, -12.4634) -> (10.7921, -12.7214) construction
  spline S540 degree 3 poles (10.7921, -12.7214) (10.7081, -12.9794) (10.6121, -13.2314) (10.5221, -13.4894) knots 49 49 49 49 50 50 50 50
  line L1777 (10.7921, -12.7214) -> (10.7081, -12.9794) construction
  line L1778 (10.7081, -12.9794) -> (10.6121, -13.2314) construction
  line L1779 (10.6121, -13.2314) -> (10.5221, -13.4894) construction
  spline S541 degree 3 poles (10.5221, -13.4894) (10.4741, -13.6274) (10.4261, -13.7714) (10.3841, -13.9094) knots 50 50 50 50 51 51 51 51
  line L1780 (10.5221, -13.4894) -> (10.4741, -13.6274) construction
  line L1781 (10.4741, -13.6274) -> (10.4261, -13.7714) construction
  line L1782 (10.4261, -13.7714) -> (10.3841, -13.9094) construction
  spline S542 degree 3 poles (10.3841, -13.9094) (10.3655, -13.9682) (10.3342, -14.0462) (10.3107, -14.1244) knots 51 51 51 51 52 52 52 52
  line L1783 (10.3841, -13.9094) -> (10.3655, -13.9682) construction
  line L1784 (10.3655, -13.9682) -> (10.3342, -14.0462) construction
  line L1785 (10.3342, -14.0462) -> (10.3107, -14.1244) construction
  spline S543 degree 3 poles (10.3107, -14.1244) (10.302, -14.1253) (10.2927, -14.1272) (10.282, -14.1314) knots 52 52 52 52 53 53 53 53
  line L1786 (10.3107, -14.1244) -> (10.302, -14.1253) construction
  line L1787 (10.302, -14.1253) -> (10.2927, -14.1272) construction
  line L1788 (10.2927, -14.1272) -> (10.282, -14.1314) construction
  spline S544 degree 3 poles (10.282, -14.1314) (10.258, -14.1434) (10.234, -14.1914) (10.216, -14.2094) knots 53 53 53 53 54 54 54 54
  line L1789 (10.282, -14.1314) -> (10.258, -14.1434) construction
  line L1790 (10.258, -14.1434) -> (10.234, -14.1914) construction
  line L1791 (10.234, -14.1914) -> (10.216, -14.2094) construction
  spline S545 degree 3 poles (10.216, -14.2094) (10.126, -14.3354) (10.036, -14.4614) (9.94, -14.5874) knots 54 54 54 54 55 55 55 55
  line L1792 (10.216, -14.2094) -> (10.126, -14.3354) construction
  line L1793 (10.126, -14.3354) -> (10.036, -14.4614) construction
  line L1794 (10.036, -14.4614) -> (9.94, -14.5874) construction
  spline S546 degree 3 poles (9.94, -14.5874) (9.724, -14.8873) (9.508, -15.1933) (9.2861, -15.4933) knots 55 55 55 55 56 56 56 56